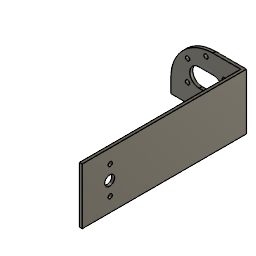
SUPPORT1 (Autodesk Fusion 360 design; units mm, degrees)
Autodesk Fusion 360 part; units mm, degrees
sketch "Esquisse1" plane through (0, 0, 0) normal (1, 0, 0) x (0, 1, 0)
  line L0 (-100, 50) -> (0, 50)
  line L1 (0, 50) -> (0, -50)
  line L2 (0, -50) -> (-100, -50)
  line L3 (-100, -50) -> (-100, 50)
  constraint horizontal L0
  constraint vertical L1
  constraint horizontal L2
  constraint vertical L3
extrude "Extrusion1" add sketch "Esquisse1" along normal blind 5 contours L0 L1 L2 L3 picked at (-66.666667, 16.666667) makes body 1
sketch "Esquisse2" plane through (5, 0, 0) normal (1, 0, 0) x (0, 1, 0)
sketch "Esquisse3" plane through (0, 0, 0) normal (1, 0, 0) x (0, 1, 0)
  line L0 (-130, 80) -> (0, 80)
  line L1 (0, 80) -> (0, 20)
  line L2 (0, 20) -> (-130, 20)
  line L3 (-130, 20) -> (-130, 80)
  constraint horizontal L0
  constraint vertical L1
  constraint horizontal L2
  constraint vertical L3
extrude "Extrusion2" add sketch "Esquisse3" against normal blind 2 contours L0 L1 L2 L3 picked at (-86.666667, 40) bodies 1
sketch "Esquisse4" plane through (0, 0, 0) normal (1, 0, 0) x (0, 1, 0)
  line L0 (0, 80) -> (2.140063, 80)
  line L1 (2.140063, 80) -> (2.140063, 20)
  line L2 (2.140063, 20) -> (0, 20)
  line L3 (0, 20) -> (0, 80)
  point P0 (0, 80)
  constraint horizontal L0
  constraint vertical L1
  constraint horizontal L2
  constraint vertical L3
  constraint coincident P0 L0.start
extrude "Extrusion3" add sketch "Esquisse4" along normal blind 0 and the other way blind 40 contours L0 L1 L2 L3 picked at (0.713354, 60) bodies 1
hole "Perçage1" at (-9.705102, 2.140063, 50) direction (0, -1, 0) diameter 13 depth 20 tip angle 118 bodies 1
hole "Perçage2" at (-20, 2.140063, 50) direction (0, -1, 0) diameter 13 depth 20 tip angle 118 bodies 1
hole "Perçage3" at (-14.264271, 2.140063, 50.148858) direction (0, -1, 0) diameter 13 depth 20 tip angle 118 bodies 1
sketch "Esquisse5" plane through (0, 0, 0) normal (0, 1, 0) x (1, 0, 0)
  circle A0 centre (-15, -50) radius 15
  line L0 (-15, -35.000001) -> (-15, -65.000001)
  line L1 (-15, -50) -> (-4.548784, -39.240257)
  line L2 (-15, -50) -> (-4.240257, -60.451216)
  line L3 (-4.240257, -60.451216) -> (-15, -50)
  line L4 (-25.759743, -39.548784) -> (-15, -50)
  line L5 (-15, -50) -> (-25.666106, -60.546762)
  dimension "d18" = 30
  constraint vertical L0
  constraint coincident A0.centre L1.start
  constraint perpendicular L1 L2
  constraint perpendicular L1 L4
  measures "d18" diameter of A0
hole "Perçage4" at (-15, 0, 35.000001) at (-25.759743, 0, 39.548784) at (-4.548784, 0, 39.240257) at (-4.240257, 0, 60.451216) at (-15, 0, 65.000001) at (-25.666106, 0, 60.546762) direction (0, 1, 0) diameter 2 depth 20 tip angle 118 bodies 1
sketch "Esquisse6" plane through (0, 0, 0) normal (0, 1, 0) x (1, 0, 0)
  line L0 (-19.832285, -43.446766) -> (-10, -43.446766)
  line L1 (-10, -43.446766) -> (-13, -49.000001)
  line L2 (-13, -49.000001) -> (-19.832285, -43.446766)
  constraint horizontal L0
extrude "Extrusion4" cut sketch "Esquisse6" along normal blind 5 contours L0 L1 L2 picked at (-14.277428, -45.297844) bodies 1
sketch "Esquisse7" plane through (0, 2.140063, 0) normal (0, 1, 0) x (-1, 0, 0)
  line L0 (0, 80) -> (0, 20)
  line L1 (0, 20) -> (40, 20)
  line L2 (40, 20) -> (40, 80)
  line L3 (40, 80) -> (0, 80)
  line L4 (19.7614, 43.504381) -> (19.832285, 43.446766)
  line L5 (19.832285, 43.446766) -> (10, 43.446766)
  line L6 (10, 43.446766) -> (10.033236, 43.508288)
  arc A0 (11.78606, 56.15789) -> (10.033236, 43.508288) centre (9.705102, 50) ccw
  arc A1 (17.283458, 55.905116) -> (11.78606, 56.15789) centre (14.264271, 50.148858) ccw
  arc A2 (19.7614, 43.504381) -> (17.283458, 55.905116) centre (20, 50) ccw
  circle A3 centre (25.666106, 60.546762) radius 1
  circle A4 centre (4.240257, 60.451216) radius 1
  circle A5 centre (25.759743, 39.548784) radius 1
  circle A6 centre (15, 35.000001) radius 1
  circle A7 centre (4.548784, 39.240257) radius 1
  circle A8 centre (15, 65.000001) radius 1
  line L7 (20.164244, 56.497925) -> (9.706392, 56.5)
  line L8 (20.164244, 56.497925) -> (9.705102, 47.681972)
  line L9 (9.705102, 47.681972) -> (9.705121, 47.77901)
  line L10 (9.706392, 56.5) -> (9.705102, 47.681972)
  constraint tangent A0 L7
  constraint perpendicular L7 L9
extrude "Extrusion5" cut sketch "Esquisse7" against normal blind 10 contours A1 A2 L7 picked at (17.382464, 56.091426) bodies 1
sketch "Esquisse8" plane through (0, 2.140063, 0) normal (0, 1, 0) x (-1, 0, 0)
  line L0 (15.652789, 56.49882) -> (19.838335, 56.497989)
  arc A0 (19.7614, 43.504381) -> (19.838335, 56.497989) centre (20, 50) ccw
  line L1 (19.7614, 43.504381) -> (19.832285, 43.446766)
  line L2 (19.832285, 43.446766) -> (10, 43.446766)
  line L3 (10, 43.446766) -> (10.033236, 43.508288)
  arc A1 (11.78606, 56.15789) -> (10.033236, 43.508288) centre (9.705102, 50) ccw
  arc A2 (15.652789, 56.49882) -> (11.78606, 56.15789) centre (14.264271, 50.148858) ccw
  line L4 (0, 80) -> (0, 20)
  line L5 (0, 20) -> (40, 20)
  line L6 (40, 20) -> (40, 80)
  line L7 (40, 80) -> (0, 80)
  circle A3 centre (25.666106, 60.546762) radius 1
  circle A4 centre (4.240257, 60.451216) radius 1
  circle A5 centre (25.759743, 39.548784) radius 1
  circle A6 centre (15, 35.000001) radius 1
  circle A7 centre (4.548784, 39.240257) radius 1
  circle A8 centre (15, 65.000001) radius 1
  line L8 (19.838335, 56.497989) -> (19.7614, 56.497989)
  line L9 (19.7614, 56.497989) -> (19.7614, 43.504381)
  line L10 (19.7614, 43.504381) -> (19.838335, 43.504381)
  line L11 (19.838335, 43.504381) -> (19.838335, 56.497989)
  line L12 (10, 43.446766) -> (19.7614, 43.446766)
  line L13 (19.7614, 43.446766) -> (19.7614, 56.497989)
  line L14 (19.7614, 56.497989) -> (10, 56.497989)
  line L15 (10, 56.497989) -> (10, 43.446766)
  constraint horizontal L8
  constraint vertical L9
  constraint horizontal L10
  constraint vertical L11
  constraint horizontal L12
  constraint vertical L13
  constraint horizontal L14
  constraint vertical L15
extrude "Extrusion6" cut sketch "Esquisse8" against normal blind 10 contours A1 A2 L14 L15 picked at (11.709766, 56.258508) bodies 1
delete_face "DeleteFace1" 1 faces at (0, -66.666667, -3.333333) on bodies 1
extrude "Extrusion7" cut 1 faces at (5, -66.666667, 30) along direction (-1, 0, 0) blind 5 on bodies 1 bodies 1
extrude "Extrusion8" add 1 faces at (0, -85.953312, 60) along direction (1, 0, 0) blind 2 on bodies 1 bodies 1
extrude "Extrusion9" cut 1 faces at (-2, -86.666667, 40) along direction (1, 0, 0) blind 2 on bodies 1 bodies 1
sketch "Esquisse9" plane through (0, 2.140063, 0) normal (0, 1, 0) x (-1, 0, 0)
  line L0 (10, 56.497989) -> (12.87196, 56.497989)
  arc A0 (15.652789, 56.49882) -> (12.87196, 56.497989) centre (14.264271, 50.148858) ccw
  line L1 (15.652789, 56.49882) -> (19.838335, 56.497989)
  arc A1 (19.7614, 43.504381) -> (19.838335, 56.497989) centre (20, 50) ccw
  line L2 (19.7614, 43.504381) -> (19.832285, 43.446766)
  line L3 (19.832285, 43.446766) -> (10, 43.446766)
  line L4 (10, 43.446766) -> (10.033236, 43.508288)
  arc A2 (10, 56.493307) -> (10.033236, 43.508288) centre (9.705102, 50) ccw
  line L5 (10, 56.493307) -> (10, 56.497989)
  line L6 (-2, 20) -> (40, 20)
  line L7 (40, 20) -> (40, 80)
  line L8 (40, 80) -> (-2, 80)
  line L9 (-2, 80) -> (-2, 20)
  circle A3 centre (25.666106, 60.546762) radius 1
  circle A4 centre (4.240257, 60.451216) radius 1
  circle A5 centre (25.759743, 39.548784) radius 1
  circle A6 centre (15, 35.000001) radius 1
  circle A7 centre (4.548784, 39.240257) radius 1
  circle A8 centre (15, 65.000001) radius 1
sketch "Esquisse10" plane through (0, 0, 0) normal (-1, 0, 0) x (0, -1, 0)
  line L0 (0, 20) -> (130, 20)
  line L1 (130, 20) -> (130, 80)
  line L2 (130, 80) -> (0, 80)
  line L3 (0, 80) -> (0, 20)
  line L4 (130, 20) -> (100, 20)
  line L5 (100, 20) -> (100, 80)
  line L6 (100, 80) -> (130, 80)
  line L7 (130, 80) -> (130, 20)
  line L8 (100, 50) -> (130, 50)
  line L9 (130, 50) -> (130, 40)
  line L10 (130, 40) -> (100, 40)
  line L11 (100, 40) -> (100, 50)
  line L12 (130, 60) -> (100, 60)
  line L13 (100, 60) -> (100, 50)
  line L14 (100, 50) -> (130, 50)
  line L15 (130, 50) -> (130, 60)
  constraint horizontal L4
  constraint vertical L5
  constraint horizontal L6
  constraint vertical L7
  constraint coincident L2 L5.end
  constraint coincident L0.end L1.start
  constraint horizontal L8
  constraint vertical L9
  constraint horizontal L10
  constraint vertical L11
  constraint coincident L7 L9.end
  constraint midpoint L5 L8.start
  constraint horizontal L12
  constraint vertical L13
  constraint horizontal L14
  constraint vertical L15
  constraint coincident L7 L12.start
hole "Perçage5" at (0, -99.993733, 40.078152) direction (1, 0, 0) diameter 3 depth 10 tip angle 118 bodies 1
hole "Perçage6" at (0, -100, 60) direction (1, 0, 0) diameter 3 depth 3 tip angle 118 bodies 1
hole "Perçage7" at (-25.759743, 2.140063, 39.548784) direction (0, -1, 0) diameter 3 depth 3 tip angle 118 bodies 1
hole "Perçage8" at (-25.666106, 2.140063, 60.546762) direction (0, -1, 0) diameter 3 depth 3 tip angle 118 bodies 1
hole "Perçage9" at (-4.240257, 2.140063, 60.451216) direction (0, -1, 0) diameter 3 depth 3 tip angle 118 bodies 1
hole "Perçage10" at (-4.548784, 2.140063, 39.240257) direction (0, -1, 0) diameter 3 depth 3 tip angle 118 bodies 1
hole "Perçage11" at (-15, 2.140063, 35.000001) direction (0, -1, 0) diameter 3 depth 3 tip angle 118 bodies 1
hole "Perçage12" at (-15, 2.140063, 65.000001) direction (0, -1, 0) diameter 3 depth 3 tip angle 118 bodies 1
sketch "Esquisse11" plane through (0, 0, 80) normal (0, 0, 1) x (-1, 0, 0)
  line L0 (0, 0) -> (0, 130)
  line L1 (0, 130) -> (-2, 130)
  line L2 (-2, 130) -> (-2, -2.140063)
  line L3 (-2, -2.140063) -> (40, -2.140063)
  line L4 (40, -2.140063) -> (40, 0)
  line L5 (40, 0) -> (0, 0)
  line L6 (0, 100) -> (100.129776, 100)
  line L7 (100.129776, 100) -> (100.129776, 0)
  line L8 (100.129776, 0) -> (0, 0)
  line L9 (0, 0) -> (0, 100)
  line L10 (10, 130) -> (100.129776, 130)
  line L11 (100.129776, 130) -> (100.129776, 70.358289)
  line L12 (100.129776, 70.358289) -> (10, 70.358289)
  line L13 (10, 70.358289) -> (10, 130)
  constraint horizontal L6
  constraint vertical L7
  constraint horizontal L8
  constraint vertical L9
  constraint coincident L0 L6.start
  constraint horizontal L10
  constraint vertical L11
  constraint horizontal L12
  constraint vertical L13
extrude "Extrusion10" add sketch "Esquisse11" along normal blind 2 separate body contours L6 L10 L11 L13 | L6 L7 L11 L12 L13 picked at (40.043259, 120) picked at (70.086517, 80.238859) makes body 2
sketch "Esquisse12" plane through (0, -70.358289, 0) normal (0, 1, 0) x (-1, 0, 0)
  line L0 (10, 80) -> (100.129776, 80)
  line L1 (100.129776, 80) -> (100.129776, 82)
  line L2 (100.129776, 82) -> (10, 82)
  line L3 (10, 82) -> (10, 80)
  line L4 (100, 20) -> (98, 20)
  line L5 (98, 20) -> (98, 80)
  line L6 (98, 80) -> (100, 80)
  line L7 (100, 80) -> (100, 20)
  dimension "d60" = 2
  constraint horizontal L4
  constraint vertical L5
  constraint horizontal L6
  constraint vertical L7
  measures "d60" distance of L4.start L4.end
extrude "Extrusion11" add sketch "Esquisse12" against normal blind 60 contours L0 L4 L5 L6 L7 picked at (98.666667, 40) bodies 2
sketch "Esquisse13" plane through (-10, 0, 0) normal (1, 0, 0) x (0, 1, 0)
  line L0 (-130, 80) -> (-70.358289, 80)
  line L1 (-70.358289, 80) -> (-70.358289, 82)
  line L2 (-70.358289, 82) -> (-130, 82)
  line L3 (-130, 82) -> (-130, 80)
  line L4 (-70.358289, 82) -> (-130.367833, 82)
  line L5 (-130.367833, 82) -> (-130.367833, 20.33491)
  line L6 (-130.367833, 20.33491) -> (-70.358289, 20.33491)
  line L7 (-70.358289, 20.33491) -> (-70.358289, 82)
  constraint horizontal L4
  constraint vertical L5
  constraint horizontal L6
  constraint vertical L7
extrude "Extrusion12" add sketch "Esquisse13" against normal blind 2 contours L0 L3 L4 L5 L6 L7 picked at (-110.242041, 40.223273) bodies 2
sketch "Esquisse14" plane through (0, -130.367833, 0) normal (0, -1, 0) x (1, 0, 0)
hole "Perçage13" at (-10, -100.363066, 35.836938) direction (-1, 0, 0) diameter 13 depth 3 tip angle 118 bodies 2
hole "Perçage14" at (-10, -100.363061, 51.167455) direction (-1, 0, 0) diameter 13 depth 3 tip angle 118 bodies 2
hole "Perçage15" at (-10, -100.363062, 43.365609) direction (-1, 0, 0) diameter 13 depth 3 tip angle 118 bodies 2
sketch "Esquisse15" plane through (-10, 0, 0) normal (1, 0, 0) x (0, 1, 0)
  arc A0 (-105.562369, 47.266533) -> (-105.6621, 39.601276) centre (-100.363062, 43.365609) ccw
  arc A1 (-95.163754, 47.266531) -> (-105.562369, 47.266533) centre (-100.363061, 51.167455) ccw
  arc A2 (-95.064029, 39.601271) -> (-95.163754, 47.266531) centre (-100.363062, 43.365609) ccw
  arc A3 (-105.6621, 39.601276) -> (-95.064029, 39.601271) centre (-100.363066, 35.836938) ccw
  line L0 (-70.358289, 20.33491) -> (-70.358289, 82)
  line L1 (-70.358289, 82) -> (-130.367833, 82)
  line L2 (-130.367833, 82) -> (-130.367833, 20.33491)
  line L3 (-130.367833, 20.33491) -> (-70.358289, 20.33491)
  line L4 (-106.862353, 51.263369) -> (-93.976281, 51.263369)
  line L5 (-93.976281, 51.263369) -> (-93.976281, 34.629053)
  line L6 (-93.976281, 34.629053) -> (-106.862353, 34.629053)
  line L7 (-106.862353, 34.629053) -> (-106.862353, 51.263369)
  constraint horizontal L4
  constraint vertical L5
  constraint horizontal L6
  constraint vertical L7
extrude "Extrusion13" cut sketch "Esquisse15" against normal blind 5 contours A0 A1 L7 | A0 A3 L7 | A1 A2 L5 | A2 A3 L5 picked at (-105.861236, 47.266539) picked at (-105.938306, 39.601289) picked at (-94.890009, 47.266531) picked at (-94.741292, 39.60127) bodies 2
sketch "Esquisse16" plane through (0, -130.367833, 0) normal (0, -1, 0) x (1, 0, 0)
hole "Perçage16" at (-100, -100.358289, 50) direction (1, 0, 0) diameter 3 depth 3 tip angle 118 bodies 2
hole "Perçage17" at (-98, -100.363069, 35.358243) direction (-1, 0, 0) diameter 3 depth 3 tip angle 118 bodies 2
hole "Perçage18" at (-100, -100.310935, 64.238032) direction (1, 0, 0) diameter 3 depth 20 tip angle 118 bodies 2
sketch "Esquisse17" plane through (0, 0, 0) normal (1, 0, 0) x (0, 1, 0)
hole "Perçage19" at (-10, -110.803509, 53.271384) direction (-1, 0, 0) diameter 3 depth 5 tip angle 118 bodies 2
hole "Perçage20" at (-10, -89.902029, 53.225904) direction (-1, 0, 0) diameter 3 depth 5 tip angle 118 bodies 2
hole "Perçage21" at (-10, -85.368309, 42.655087) direction (-1, 0, 0) diameter 3 depth 5 tip angle 118 bodies 2
hole "Perçage22" at (-10, -89.902039, 31.754122) direction (-1, 0, 0) diameter 3 depth 5 tip angle 118 bodies 2
hole "Perçage23" at (-10, -110.914011, 31.818943) direction (-1, 0, 0) diameter 3 depth 5 tip angle 118 bodies 2
hole "Perçage24" at (-10, -115.365143, 42.649188) direction (-1, 0, 0) diameter 3 depth 5 tip angle 118 bodies 2
hole "Perçage25" at (2, -100.372475, 49.984168) direction (-1, 0, 0) diameter 7 depth 3 tip angle 118 bodies 1
move_body "Déplacer1" bodies 2 to x (1, 0, 0) y (0, 1, 0) z (0, 0, 1) at (5, 0, 0)
delete_body "RemoveBody1" bodies 2
move_face "DéplacerFace1" by (0, -5, 0) 1 faces at (-35.499962, 0, 49.987171) on bodies 1
move_face "DéplacerFace2" by (0, -5, 0) 1 faces at (-35.499962, 2.140063, 49.987171) on bodies 1
sketch "Esquisse18" plane through (0, 0, 0) normal (0, 1, 0) x (1, 0, 0)
move_face "DéplacerFace3" to x (1, 0, 0) y (0, 1, 0) z (0, 0, 1) at (0.02934, 0, 0.499138) 1 faces at (-16.124672, -3.573291, 65.99253) on bodies 1
move_face "DéplacerFace4" to x (0.9961947, 0, -0.08715574) y (0, 1, 0) z (0.08715574, 0, 0.9961947) at (-3.121808, 0, -1.673947) 1 faces at (-13.665193, -4.286646, 34.315685) on bodies 1
move_face "DéplacerFace5" to x (1, 0, 0) y (0, 1, 0) z (0, 0, 1) at (0.363503, 0, -0.343316) 1 faces at (-4.474015, -3.573291, 40.738392) on bodies 1
move_face "DéplacerFace6" to x (1, 0, 0) y (0, 1, 0) z (0, 0, 1) at (-0.343315, 0, -0.363503) 1 faces at (-24.424936, -4.286646, 38.864468) on bodies 1
move_face "DéplacerFace7" to x (1, 0, 0) y (0, 1, 0) z (0, 0, 1) at (0.321394, 0, 0.383022) 1 faces at (-4.165488, -3.573291, 61.949352) on bodies 1
move_face "DéplacerFace8" to x (1, 0, 0) y (0, 1, 0) z (0, 0, 1) at (-0.321394, 0, 0.383022) 1 faces at (-24.331298, -4.286646, 59.862446) on bodies 1
move_face "DéplacerFace9" to x (1, 0, 0) y (0, 1, 0) z (0, 0, 1) at (1.491819, 0, -2.00611) 1 faces at (-2.584055, -4.286646, 60.149923) on bodies 1
move_face "DéplacerFace10" to x (1, 0, 0) y (0, 1, 0) z (0, 0, 1) at (-1.491829, 0, -2.006102) 1 faces at (-27.431436, -3.573291, 61.336045) on bodies 1
move_face "DéplacerFace11" to x (1, 0, 0) y (0, 1, 0) z (0, 0, 1) at (1.716576, 0, 1.817517) 1 faces at (-4.110512, -3.573291, 40.395076) on bodies 1
move_face "DéplacerFace12" to x (1, 0, 0) y (0, 1, 0) z (0, 0, 1) at (-1.817516, 0, 1.716576) 1 faces at (-24.768251, -4.286646, 38.500964) on bodies 1
sketch "Esquisse19" plane through (0, 0, 0) normal (0, 1, 0) x (1, 0, 0)
move_face "DéplacerFace13" to x (1, 0, 0) y (0, 1, 0) z (0, 0, 1) at (-2.078461, 0, -1.199999) 1 faces at (-26.144521, -4.286646, 58.239366) on bodies 1
move_face "DéplacerFace14" to x (1, 0, 0) y (0, 1, 0) z (0, 0, 1) at (1.542689, 0, -1.838508) 1 faces at (-2.352275, -3.573291, 60.326264) on bodies 1
move_face "DéplacerFace15" to x (1, 0, 0) y (0, 1, 0) z (0, 0, 1) at (1.542691, 0, 1.838506) 1 faces at (-2.393936, -3.573291, 42.212593) on bodies 1
move_face "DéplacerFace16" to x (1, 0, 0) y (0, 1, 0) z (0, 0, 1) at (-1.199998, 0, 2.078462) 1 faces at (-26.585767, -4.286646, 40.217541) on bodies 1
move_face "DéplacerFace17" to x (1, 0, 0) y (0, 1, 0) z (0, 0, 1) at (1, 0, -0.000001) 1 faces at (-27.785765, -4.286646, 42.296003) on bodies 1
move_face "DéplacerFace18" to x (1, 0, 0) y (0, 1, 0) z (0, 0, 1) at (1, 0, 0) 1 faces at (-31.001727, -3.573291, 58.129943) on bodies 1
move_face "DéplacerFace19" to x (0.98480775, 0, -0.17364818) y (0, 1, 0) z (0.17364818, 0, 0.98480775) at (-10.909579, 0, 0.712234) 1 faces at (-1.820375, -3.573291, 55.8175) on bodies 1
move_face "DéplacerFace20" to x (1, 0, 0) y (0, 1, 0) z (0, 0, 1) at (-1, 0, 0) 1 faces at (-0.378692, -3.573291, 41.156382) on bodies 1
sketch "Esquisse20" plane through (0, 0, 0) normal (0, 1, 0) x (1, 0, 0)
move_face "DéplacerFace21" to x (0.9961947, 0, -0.08715574) y (0, 1, 0) z (0.08715574, 0, 0.9961947) at (-4.988419, 0, 0.552427) 1 faces at (-0.430739, -3.573291, 57.359758) on bodies 1
move_face "DéplacerFace22" to x (0.98480775, 0, 0.17364818) y (0, 1, 0) z (-0.17364818, 0, 0.98480775) at (5.748522, 0, 3.631134) 1 faces at (-14.809222, -3.573291, 35.986122) on bodies 1
move_face "DéplacerFace23" to x (0.90630779, 0, 0.42261826) y (0, 1, 0) z (-0.42261826, 0, 0.90630779) at (22.219236, 0, 17.463026) 1 faces at (-30.001727, -3.573291, 58.129943) on bodies 1
extrude "Extrusion14" add 1 faces at (2, -34.200712, 50.081908) along direction (1, 0, 0) blind 9.8 on bodies 1 bodies 1
extrude "Extrusion15" cut 1 faces at (0, -35.62742, 50.081908) along direction (1, 0, 0) blind 9.8 on bodies 1 bodies 1
extrude "Extrusion16" cut 1 faces at (-6.133333, -3.573291, 80) along direction (0, 0, -1) blind 10 on bodies 1 bodies 1
fillet "Congé1" radius 30 1 edges at (-40, -3.929968, 70) on bodies 1
extrude "Extrusion17" cut 1 faces at (10.466667, -130, 36.666667) along direction (0, 1, 0) blind 10 on bodies 1 bodies 1
extrude "Extrusion18" cut 1 faces at (-6.133333, -3.573291, 20) along direction (0, 0, 1) blind 10 on bodies 1 bodies 1
sketch "Esquisse21" plane through (-0.011212, 0, 56.501924) normal (0.000198, 0, -1) x (0, 1, 0)
  line L0 (-5, -15.641577) -> (-5, -19.827123)
  line L1 (-5, -19.827123) -> (-2.859937, -19.827123)
  line L2 (-2.859937, -19.827123) -> (-2.859937, -15.641577)
  line L3 (-2.859937, -15.641577) -> (-5, -15.641577)
  line L4 (-5, -12.860748, 0.001382) -> (-5, -15.641577, 0)
  line L5 (-2.859937, -15.641577) -> (-5, -15.641577)
  line L6 (-5, -15.641577) -> (-5, -13)
  line L7 (-5, -13) -> (-2.859937, -13)
  line L8 (-2.859937, -13) -> (-2.859937, -15.641577)
  point P0 (-5, -12.860748)
  constraint vertical L6
  constraint perpendicular L5 L6
  constraint horizontal L7
  constraint parallel L6 L8
extrude "Extrusion19" add sketch "Esquisse21" against normal blind 2 contours L3 L5 L6 L7 L8 picked at (-4.286646, -13.880526) bodies 1
sketch "Esquisse22" plane through (-0.011212, 0, 56.501924) normal (0.000198, 0, -1) x (0, 1, 0)
  line L0 (-5, -13) -> (-5, -19.827123)
  line L1 (-5, -19.827123) -> (-2.859937, -19.827123)
  line L2 (-2.859937, -19.827123) -> (-2.859937, -13)
  line L3 (-2.859937, -13) -> (-5, -13)
